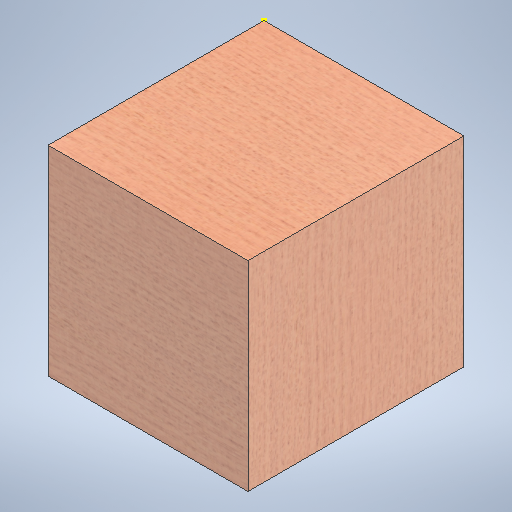
# Autodesk Inventor part: Caja grande
Saved by Autodesk Inventor 2025.1 (Build 291241000, 241)
## iProperties
Created: 2025-02-26
Part Number: Caja grande
Material: Generic
Document SubType Name: Modeling
Designer: yovan
Density: 1 g/cm^3
Appearance: Default
Author: yovan
Autodesk Inventor part; units mm, degrees
ref_plane "YZ Plane" through (0, 0, 0) normal (1, 0, 0) x (0, 1, 0)
ref_plane "XZ Plane" through (0, 0, 0) normal (0, 1, 0) x (-1, 0, 0)
ref_plane "XY Plane" through (0, 0, 0) normal (0, 0, 1) x (1, 0, 0)
sketch "Sketch1" plane through (0, 0, 0) normal (1, 0, 0) x (0, 1, 0)
  line L0 (0, 0) -> (250, 0)
  line L1 (250, 0) -> (250, 270)
  line L2 (250, 270) -> (0, 270)
  line L3 (0, 270) -> (0, 0)
  dimension "d0" = 250
  dimension "d1" = 270
  constraints: 8 end point, 2 parallel, 1 horizontal, 1 perpendicular
  measures "d0" distance of L2.end L1.end
  measures "d1" distance of L1.end L0.end
extrude "Extrusion1" add sketch "Sketch1" along normal blind 250
shell "Shell1" thickness 2 removed faces 1 at (166.6667, 166.6667, 270)
sketch "Sketch2" plane through (0, 250, 270) normal (0, 1, 0) x (1, 0, 0)
  point P0 (0, 270)
sketch "Sketch3" plane through (2, 248, 2) normal (0, -1, 0) x (1, 0, 0)
  line L0 (0, 268) -> (246, 268) projected
  line L1 (0, 268) -> (246, 268)
  line L2 (246, 268) -> (246, 266)
  line L3 (246, 266) -> (0, 266)
  line L4 (0, 266) -> (0, 268)
  point P0 (-2, -2)
  dimension "d5" = 246
  dimension "d6" = 2
  constraints: 8 end point, 2 parallel, 1 horizontal, 1 perpendicular
  measures "d5" distance of L2.end L3.end
  measures "d6" distance of L1.end L2.end
extrude "Extrusion2" add sketch "Sketch3" along normal blind 246
body "Solid1"
